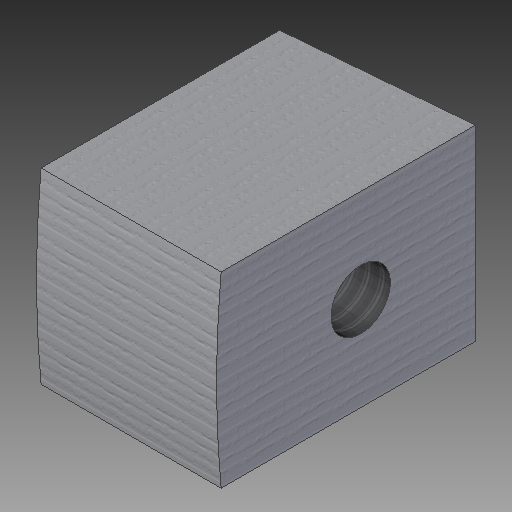
# Autodesk Inventor part: 32110_Lock Wedge_V1
Saved by Autodesk Inventor 2020 (Build 240168000, 168)
## iProperties
Created: 2018-11-30
Part Number: 32110_Lock Wedge_V1
Material: Acetal Resin, White
Document SubType Name: Modeling
Designer: MPI
Density: 1.425 g/cm^3
Appearance: Smooth - White
Mass: 1.93112 g
Surface Area: 8.57058 cm^2
Volume: 1.35517 cm^3
Author: MPI
Autodesk Inventor part; units mm, degrees
ref_plane "YZ Plane" through (0, 0, 0) normal (1, 0, 0) x (0, 1, 0)
ref_plane "XZ Plane" through (0, 0, 0) normal (0, 1, 0) x (-1, 0, 0)
ref_plane "XY Plane" through (0, 0, 0) normal (0, 0, 1) x (1, 0, 0)
sketch "Sketch1" plane through (0, 0, 0) normal (1, 0, 0) x (0, 1, 0)
  circle A0 centre (0, 0) radius 54
  circle A1 centre (0, 46) radius 1
  circle A2 centre (0, 46) radius 5.5
  line L0 (5.2, 40.5) -> (-5.2, 40.5)
  arc A3 (5.2, 53.749) -> (-5.2, 53.749) centre (0, 0) ccw
  line L1 (5.2, 53.749) -> (5.2, 40.5)
  line L2 (-5.2, 53.749) -> (-5.2, 40.5)
  circle A4 centre (0, 46) radius 5.2
  dimension "d0" = 108
  dimension "d1" = 46
  dimension "d2" = 2
  dimension "d3" = 11
  dimension "d23" = 10.4
  dimension "d24" = 0
  constraints: 6 end point, 5 centre point, 4 point on circle, 3 coincident, 3 tangent, 1 concentric, 1 horizontal
  measures "d0" diameter of A0
  measures "d1" distance of A1.centre A0.centre
  measures "d2" diameter of A1
  measures "d3" diameter of A2
  measures "d23" diameter of A4
  measures "d24" horizontal distance of point (0, 0) A1.centre
extrude "Extrusion1" add sketch "Sketch1" along normal blind 10 contours L1 A2 L2 A0 | L1 A4 L2 A2 | A4 | L1 A2 L2 A4 | A2 L0 L2 | L1 L0 A2 | A1
sketch "Sketch2" plane through (10, 0, 0) normal (1, 0, 0) x (0, 0, -1)
  circle A0 centre (0, 0) radius 54
  point P0 (-46, 0)
  dimension "d15" = 46
  constraints: 1 centre point, 1 coincident
  measures "d15" distance of point (0, 0) point (-46, 0)
hole "Hole2" at (10, 0, 46) direction (-1, 0, 0) diameter 3.302 end through all thread size "8-32 UNC" class "2B" standard "ANSI Unified Screw Threads"
sketch "Sketch3" plane through (0, -5.2, 40.5) normal (0, -1, 0) x (1, 0, 0)
  line L0 (0, 0) -> (10, 0)
  line L1 (0, 0) -> (10, 0) projected
  line L2 (10.0706, -0.8811) -> (0, 0)
  line L3 (10, 13.249) -> (10, 0) projected
  line L4 (10, 0) -> (10, -0.8749)
  point P0 (0, -40.5)
  dimension "d25" = 5
  constraints: 6 end point, 1 collinear, 1 horizontal, 1 point on line
  measures "d25" angle of L2 L0
extrude "Extrusion2" add sketch "Sketch3" against normal up to surface (10.4 mm away)
body "Solid1"
